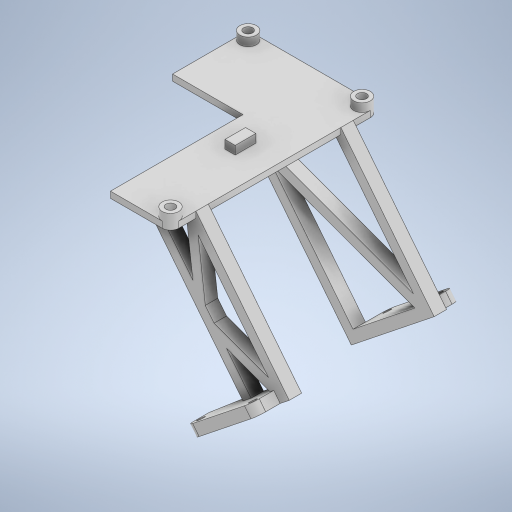
# Autodesk Inventor part: Base_ScreenHolder
Saved by Autodesk Inventor 2023 (Build 270158000, 158)
## iProperties
Created: 2025-02-11
Part Number: Base_ScreenHolder
Material: Generic
Document SubType Name: Modeling
Designer: Swoby
Density: 1 g/cm^3
Appearance: Default
Author: Swoby
Autodesk Inventor part; units mm, degrees
ref_plane "YZ Plane" through (0, 0, 0) normal (1, 0, 0) x (0, 1, 0)
ref_plane "XZ Plane" through (0, 0, 0) normal (0, 1, 0) x (-1, 0, 0)
sketch "Sketch1" plane through (0, 0, 0) normal (0, 1, 0) x (-1, 0, 0)
  line L0 (-27.5, 46.25) -> (27.5, 46.25) construction
  line L1 (27.5, 46.25) -> (27.5, -46.25) construction
  line L2 (27.5, -46.25) -> (-27.5, -46.25) construction
  line L3 (-27.5, -46.25) -> (-27.5, 46.25) construction
  line L4 (-27.5, 46.25) -> (27.5, -46.25) construction
  line L5 (27.5, 46.25) -> (-27.5, -46.25) construction
  line L6 (-2.5, 46.25) -> (-2.5, -13.75)
  line L7 (-2.5, -13.75) -> (27.5, -13.75)
  circle A0 centre (-27.5, 46.25) radius 2.15
  circle A1 centre (27.5, -46.25) radius 2.15
  circle A2 centre (-27.5, -46.25) radius 2.15
  line L8 (-27.5, 50.25) -> (-2.5, 50.25)
  line L9 (-2.5, 50.25) -> (-2.5, 46.25)
  line L10 (-31.5, 46.25) -> (-31.5, -46.25)
  line L11 (-27.5, -50.25) -> (27.5, -50.25)
  line L12 (27.5, -13.75) -> (31.5, -13.75)
  line L13 (31.5, -13.75) -> (31.5, -46.25)
  arc A3 (-27.5, 50.25) -> (-31.5, 46.25) centre (-27.5, 46.25) ccw
  arc A4 (-31.5, -46.25) -> (-27.5, -50.25) centre (-27.5, -46.25) ccw
  arc A5 (27.5, -50.25) -> (31.5, -46.25) centre (27.5, -46.25) ccw
  point P0 (0, 0)
  dimension "d0" = 55
  dimension "d1" = 92.5
  dimension "d2" = 30
  dimension "d3" = 60
  dimension "d4" = 4.3
  dimension "d5" = 4.3
  dimension "d7" = 4.3
  dimension "d10" = 4
  dimension "d11" = 4
  dimension "d12" = 4
  constraints: 28 end point, 6 centre point, 6 coincident, 6 point on circle, 5 perpendicular, 5 tangent, 3 horizontal, 2 midpoint, 2 parallel, 2 point on line, 1 vertical
  measures "d0" distance of L1.end L2.end
  measures "d1" distance of L0.end L1.end
  measures "d2" distance between parallel lines of L6 L1
  measures "d3" distance between parallel lines of L0 L7
  measures "d4" diameter of A0
  measures "d5" diameter of A1
  measures "d7" diameter of A2
  measures "d10" radius of A3
  measures "d11" radius of A4
  measures "d12" radius of A5
extrude "Extrusion1" add sketch "Sketch1" along normal blind 3
sketch "Sketch2" plane through (0, 3, 0) normal (0, 1, 0) x (1, 0, 0)
  line L0 (31.5, -46.25) -> (31.5, 46.25) projected
  arc A0 (31.5, 46.25) -> (27.5, 50.25) centre (27.5, 46.25) ccw projected
  line L1 (27.5, 50.25) -> (-27.5, 50.25) projected
  arc A1 (-27.5, 50.25) -> (-31.5, 46.25) centre (-27.5, 46.25) ccw projected
  line L2 (-31.5, 46.25) -> (-31.5, 13.75) projected
  line L3 (-31.5, 13.75) -> (2.5, 13.75) projected
  line L4 (2.5, 13.75) -> (2.5, -50.25) projected
  line L5 (2.5, -50.25) -> (27.5, -50.25) projected
  arc A2 (27.5, -50.25) -> (31.5, -46.25) centre (27.5, -46.25) ccw projected
  circle A3 centre (27.5, 46.25) radius 2.15 projected
  circle A4 centre (-27.5, 46.25) radius 2.15 projected
  circle A5 centre (27.5, -46.25) radius 2.15 projected
  circle A6 centre (27.5, -46.25) radius 4
  circle A7 centre (27.5, 46.25) radius 4
  circle A8 centre (-27.5, 46.25) radius 4
  line L6 (27.5, -46.25) -> (27.5, 46.25) construction
  line L7 (27.5, 0) -> (15, 0) construction
  line L8 (12.5, -5) -> (17.5, -5)
  line L9 (17.5, -5) -> (17.5, 5)
  line L10 (17.5, 5) -> (12.5, 5)
  line L11 (12.5, 5) -> (12.5, -5)
  line L12 (12.5, -5) -> (17.5, 5) construction
  line L13 (17.5, -5) -> (12.5, 5) construction
  line L14 (15, 0) -> (15, -50.25) construction
  point P0 (0, 0)
  point P1 (-31.5, 46.25)
  point P2 (27.5, 50.25)
  dimension "d15" = 5
  dimension "d16" = 10
  dimension "d17" = 29
  dimension "d18" = 16.5
  constraints: 18 end point, 4 midpoint, 3 coincident, 2 horizontal, 2 parallel, 1 centre point, 1 concentric, 1 perpendicular, 1 vertical, 6 other
  measures "d15" distance of L10.end L9.end
  measures "d16" distance of L9.end L8.end
  measures "d17" distance between parallel lines of L0 L4
  measures "d18" distance between parallel lines of L0 L14
extrude "Extrusion2" add sketch "Sketch2" along normal blind 4 contours A2 A6 | A7 A0 | A8 A1 | L11 L10 L9 L8
sketch "Sketch3" plane through (27.5, 0, -50.25) normal (0, 0, -1) x (-1, 0, 0)
  line L0 (0, 0) -> (55, 0) projected
  line L1 (55, 0) -> (55, 3) projected
  line L2 (0, 3) -> (55, 3) projected
  line L3 (0, 0) -> (0, 3) projected
  line L4 (59, 0) -> (59, 3) projected
  line L5 (-4, 0) -> (-4, 3) projected
  line L6 (-4, 3) -> (-49.081, -53.5836)
  line L7 (59, 0) -> (-9.081, -85.4522)
  line L8 (-9.081, -85.4522) -> (-49.081, -53.5836)
  line L9 (59, 3) -> (55, 3)
  line L10 (0, 3) -> (-4, 3)
  line L11 (0, 0) -> (-39.065, -49.0326)
  line L12 (-42.0564, -52.7873) -> (-39.7673, -54.611) construction
  line L13 (-9.8743, -78.4273) -> (29.1908, -29.3946)
  line L14 (-21.0282, -26.3936) -> (11.1539, -52.0336) construction
  line L15 (-42.0564, -52.7873) -> (32.1821, -25.64) construction
  line L16 (29.1908, -29.3946) -> (-39.7673, -54.611)
  line L17 (35.1735, -21.8853) -> (-39.065, -49.0326)
  line L18 (35.1735, -21.8853) -> (52.6099, 0)
  line L19 (29.1908, -29.3946) -> (35.1735, -21.8853) construction
  line L20 (-39.065, -49.0326) -> (-42.0564, -52.7873) construction
  line L21 (-39.7673, -54.611) -> (-9.8743, -78.4273)
  point P0 (27.5, 0)
  point P1 (-4.9371, -39.2136)
  point P2 (-4.9371, -39.2136)
  dimension "d21" = 40
  dimension "d22" = 70
  dimension "d23" = 5
  dimension "d24" = 4.9979
  dimension "d25" = 4.9979
  dimension "d26" = 4.9979
  dimension "d27" = 2.4989
  dimension "d28" = 33.7463
  dimension "d29" = 67.4925
  dimension "d30" = 20.5736
  dimension "d31" = 41.1473
  constraints: 32 end point, 8 parallel, 8 perpendicular, 4 midpoint, 3 point on line, 1 collinear, 1 horizontal
  measures "d21" horizontal distance of L7.end L6.end
  measures "d22" distance from line of L8 L5.start
  measures "d23" distance between parallel lines of L8 L12
  measures "d24" distance between parallel lines of L6 L11
  measures "d25" distance between parallel lines of L7 L13
  measures "d26" distance between parallel lines of L16 L17
  measures "d27" distance between parallel lines of L17 L15
  measures "d28" distance from line of L12.start L14
  measures "d29" distance of L12.start L0.start
  measures "d30" distance of point (-4.937, -39.214) L14.start
  measures "d31" distance between parallel lines of L13 L11
ref_plane "Work Plane1" through (0, 0, -35) normal (0, 0, 1) x (1, 0, 0)
extrude "Extrusion3" add sketch "Sketch3" along normal mid plane 6 from surface at -15.25 contours L11 L17 L18 L0 L1 L9 L4 L7 L8 L6 L10 L3
sketch "Sketch4" plane through (67.2673, -54.611, -32) normal (-0.6231268, 0.7821208, 0) x (0.7821208, 0.6231268, 0)
  line L0 (74.1042, -32) -> (-124.8943, -32) projected
  line L1 (7.9246, 0) -> (-43.2184, 0) projected
  line L2 (-43.2184, 0) -> (-43.2184, 6) projected
  line L3 (7.9246, 6) -> (-43.2184, 6) projected
  line L4 (7.9246, 0) -> (7.9246, 6) projected
  line L5 (-17.6469, 6) -> (-17.6469, 27.9873) construction
  line L6 (-1.6469, 13) -> (-33.6469, 13) construction
  circle A0 centre (-1.6469, 13) radius 1.75
  circle A1 centre (-33.6469, 13) radius 1.75
  line L7 (-1.6469, 13) -> (-33.6469, 13) construction
  line L8 (-1.6469, 17) -> (-33.6469, 17)
  line L9 (-33.6469, 9) -> (-1.6469, 9)
  arc A2 (-1.6469, 9) -> (-1.6469, 17) centre (-1.6469, 13) ccw
  arc A3 (-33.6469, 17) -> (-33.6469, 9) centre (-33.6469, 13) ccw
  line L10 (2.3531, 13) -> (2.3531, 6)
  line L11 (-37.6469, 13) -> (-37.6469, 6)
  point P0 (-18.5816, -32)
  point P1 (-17.6469, 13)
  point P2 (-17.6469, 13)
  dimension "d35" = 32
  dimension "d36" = 3.5
  dimension "d37" = 3.5
  dimension "d38" = 90
  dimension "d39" = 8
  constraints: 16 end point, 6 point on circle, 5 tangent, 4 centre point, 3 midpoint, 3 point on line, 2 coincident, 2 equal length, 1 horizontal, 1 perpendicular, 1 vertical
  measures "d35" distance of L6.start L6.end
  measures "d36" diameter of A0
  measures "d37" diameter of A1
  measures "d38" diameter of L6 L0
  measures "d39" diameter of A3
extrude "Extrusion4" add sketch "Sketch4" against normal up to surface (5 mm away) from surface at 0 contours L3 L11 A3 L9 A2 L10 | A2 L9 A3 L8
ref_plane "Work Plane2" through (0, 0, 35) normal (0, 0, 1) x (1, 0, 0)
sketch "Sketch5" plane through (0, 0, 35) normal (0, 0, 1) x (1, 0, 0)
  line L0 (2.5, 0) -> (27.5, 0) projected
  line L1 (27.5, 0) -> (27.5, 3) projected
  line L2 (2.5, 3) -> (27.5, 3) projected
  line L3 (2.5, 0) -> (2.5, 3) projected
  line L4 (36.581, -85.4522) -> (-31.5, 0) projected
  line L5 (76.581, -53.5836) -> (36.581, -85.4522) projected
  line L6 (31.5, 3) -> (76.581, -53.5836) projected
  line L7 (31.5, 0) -> (31.5, 3) projected
  line L8 (27.5, 0) -> (31.5, 0) projected
  line L9 (66.565, -49.0326) -> (27.5, 0) projected
  line L10 (-7.6735, -21.8853) -> (66.565, -49.0326) projected
  line L11 (-25.1099, 0) -> (-7.6735, -21.8853) projected
  line L12 (-31.5, 0) -> (-25.1099, 0) projected
  line L13 (-1.6908, -29.3946) -> (37.3743, -78.4273) projected
  line L14 (67.2673, -54.611) -> (-1.6908, -29.3946) projected
  line L15 (37.3743, -78.4273) -> (67.2673, -54.611) projected
  line L16 (2.5, 0) -> (57.3792, -68.8819)
  line L17 (27.5, 3) -> (31.5, 3)
  line L18 (31.2871, -36.1323) -> (37.2699, -43.6416)
  line L19 (34.2785, -39.887) -> (29.5863, -2.6187) construction
  line L20 (34.2785, -39.887) -> (69.5564, -52.7873) construction
  line L21 (34.2785, -39.887) -> (36.5676, -38.0633) construction
  line L22 (31.2871, -36.1323) -> (30.0878, -26.6063) construction
  line L23 (36.5676, -38.0633) -> (36.0706, -34.1156) construction
  line L24 (8.8901, 0) -> (40.3044, -39.4297)
  line L25 (30.0878, -26.6063) -> (26.738, 0)
  line L26 (36.0706, -34.1156) -> (32.5777, -6.3733)
  line L27 (46.2871, -46.939) -> (58.1725, -61.857)
  line L28 (40.3044, -39.4297) -> (46.2871, -46.939) construction
  point P0 (0, 0)
  dimension "d43" = 58.631
  dimension "d44" = 58.631
  dimension "d45" = 2.4989
  dimension "d46" = 4.9979
  dimension "d47" = 2.4989
  dimension "d49" = 4.9979
  dimension "d50" = 4.9979
  constraints: 26 end point, 18 point on line, 8 parallel, 2 perpendicular, 1 horizontal, 1 midpoint
  measures "d43" angle of L20 L21
  measures "d44" angle of L19 L21
  measures "d45" distance between parallel lines of L19 L22
  measures "d46" distance between parallel lines of L14 L10
  measures "d47" distance between parallel lines of L23 L19
  measures "d49" distance between parallel lines of L6 L9
  measures "d50" distance between parallel lines of L16 L24
extrude "Extrusion5" add sketch "Sketch5" along normal mid plane 6 contours L0 L24 L10 L16 | L10 L9 L8 L7 L6 L5 L16 L15 L14 | L0 L9 L26 L24 L25 | L14 L27 L15 L16
mirror "Mirror1" about plane through (0, 0, 0) normal (0, 0, 1) of "Extrusion4"
chamfer "Chamfer1" distance 21 distance2 6 1 edges at (55.8214, -66.9266, 38) measured on face at (55.4303, -67.2382, 38)
equation "\"d25\" = d24"
equation "\"d26\" = d24"
equation "\"d27\" = 0.5 * d26"
equation "\"d28\" = 0.5 * d29"
equation "\"d30\" = 0.5 * d31"
equation "\"d44\" = d43"
equation "\"d45\" = 0.5 * d46"
equation "\"d47\" = d45"
equation "\"d50\" = d49"
body "Solid1"
